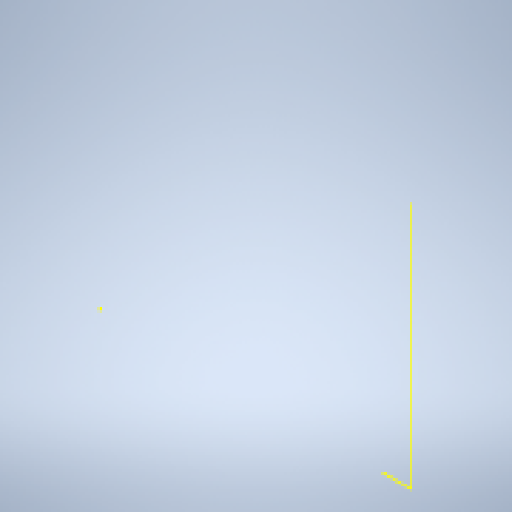
# Autodesk Inventor part: Soporte Motor
Saved by Autodesk Inventor 2024 (Build 280153000, 153)
## iProperties
Created: 2025-03-08
Part Number: Soporte Motor
Material: Genérico
Document SubType Name: Modeling
Designer: sergi
Density: 1 g/cm^3
Appearance: Valor por defecto
Author: sergi
Autodesk Inventor part; units mm, degrees
ref_plane "YZ Plane" through (0, 0, 0) normal (1, 0, 0) x (0, 1, 0)
ref_plane "XZ Plane" through (0, 0, 0) normal (0, 1, 0) x (-1, 0, 0)
ref_plane "XY Plane" through (0, 0, 0) normal (0, 0, 1) x (1, 0, 0)
sketch "Boceto1" plane through (0, 0, 0) normal (0, 0, 1) x (1, 0, 0)
  line L0 (42.301, 0) -> (42.301, 9.6) projected
  line L1 (42.302, 9.6) -> (42.302, 26.1) projected
  line L2 (42.301, 26.1) -> (42.301, 33.75) projected
  line L3 (38.301, 0) -> (42.301, 0) projected
  line L4 (4.001, 33.75) -> (38.301, 33.75) projected
  line L5 (38.301, 33.75) -> (42.301, 33.75) projected
  line L6 (0.001, 33.75) -> (4.001, 33.75) projected
  line L7 (0.001, 26.1) -> (0.001, 33.75) projected
  line L8 (0.001, 9.6) -> (0.001, 26.1) projected
  line L9 (0.001, 0) -> (0.001, 9.6) projected
  line L10 (42.301, 33.75) -> (0.001, 33.75)
  line L11 (0.001, 33.75) -> (0.001, 0)
  line L12 (0.001, 0) -> (42.301, 0)
  line L13 (42.301, 0) -> (42.301, 33.75)
  line L14 (42.501, 33.95) -> (-0.199, 33.95)
  line L15 (-0.199, 33.95) -> (-0.199, -0.2)
  line L16 (-0.199, -0.2) -> (42.501, -0.2)
  line L17 (42.501, -0.2) -> (42.501, 33.95)
  line L18 (42.501, 36.95) -> (-3.199, 36.95)
  line L19 (-3.199, 36.95) -> (-3.199, 0)
  line L20 (-3.199, -3.2) -> (45.501, -3.2)
  line L21 (45.501, 0) -> (45.501, 36.95)
  line L22 (42.301, 0) -> (45.501, 0)
  line L23 (0.001, 0) -> (-3.199, 0)
  line L24 (42.501, 33.95) -> (42.501, 36.95)
  point P0 (0, 0)
  point P1 (-0.199, 0)
  dimension "d0" = 0.2
  dimension "d1" = 3
  constraints: 30 end point, 6 parallel, 4 perpendicular, 2 point on line, 1 horizontal, 3 other
  measures "d0" distance between parallel lines of L13 L17
  measures "d1" distance between parallel lines of L17 L21
extrude "Extrusión1" add sketch "Boceto1" along normal blind 45.502 contours L14 L15 L23 L19 L18 L24
sketch "Boceto2" plane through (-0.199, 33.95, 0) normal (0, -1, 0) x (1, 0, 0)
  line L0 (0, 0) -> (42.7, 0) projected
  line L1 (42.7, 0) -> (42.7, 45.502) projected
  line L2 (0, 45.502) -> (42.7, 45.502) projected
  line L3 (0, 0) -> (0, 45.502) projected
  line L4 (42.7, 45.502) -> (0, 45.502)
  line L5 (0, 45.502) -> (0, 42.502)
  line L6 (0, 42.502) -> (42.7, 42.502)
  line L7 (42.7, 42.502) -> (42.7, 45.502)
  point P0 (0.199, 0)
  dimension "d4" = 3
  constraints: 8 end point, 2 parallel, 1 horizontal, 1 perpendicular, 1 point on line
  measures "d4" distance of L5.end L4.end
extrude "Extrusión2" add sketch "Boceto2" along normal up to surface (33.95 mm away) contours L3 L2 L1 L6
sketch "Boceto3" plane through (0, 0, 45.502) normal (0, 0, 1) x (1, 0, 0)
  line L0 (-3.199, 0) -> (42.501, 0) projected
  line L1 (42.501, 36.95) -> (42.501, 0) projected
  line L2 (42.501, 36.95) -> (-3.199, 36.95) projected
  line L3 (-3.199, 36.95) -> (-3.199, 0) projected
  line L4 (-6.5037, 43.25) -> (-6.5037, 58.25) projected
  line L5 (-6.5037, 43.25) -> (-6.5037, 58.25) projected
  line L6 (29.151, 9.6) -> (29.151, 3.2) projected
  line L7 (29.151, 0) -> (29.151, 3.2) projected
  line L8 (13.651, 3.6) -> (13.651, 9.1) projected
  line L9 (13.151, 3.2) -> (13.151, 0) projected
  line L10 (13.151, 9.6) -> (13.151, 3.2) projected
  line L11 (29.151, 9.6) -> (13.151, 9.6) projected
  line L12 (11.151, 0) -> (11.151, 3.2)
  line L13 (11.151, 3.2) -> (11.151, 11.6)
  line L14 (11.151, 11.6) -> (31.151, 11.6)
  line L15 (31.151, 11.6) -> (31.151, 3.2)
  line L16 (31.151, 3.2) -> (31.151, 0)
  point P0 (0, 0)
  point P1 (-15.9908, 43.25)
  dimension "d7" = 2
  constraints: 10 end point, 5 other
  measures "d7" distance between parallel lines of L11 L14
extrude "Extrusión3" cut sketch "Boceto3" against normal blind 10 contours L12 L13 L14 L15 L16 L0 L7 L6 L11 L10 L9 | L9 L10 L11 L6 L7 L0
sketch "Boceto4" plane through (-3.199, 36.95, 0) normal (0, 1, 0) x (1, 0, 0)
  circle A0 centre (24.35, -21.151) radius 2.5 projected
  circle A1 centre (24.35, -21.151) radius 15
  point P0 (3.199, 0)
  dimension "d10" = 30
  constraints: 1 centre point, 1 coincident
  measures "d10" diameter of A1
extrude "Extrusión4" cut sketch "Boceto4" against normal blind 10 contours A0 | A1
sketch "Boceto5" plane through (-3.199, 36.95, 0) normal (0, 1, 0) x (1, 0, 0)
  circle A0 centre (24.35, -21.151) radius 15 projected
  line L0 (45.7, 0) -> (0, 0) projected
  line L1 (0, 0) -> (0, -45.502) projected
  line L2 (45.7, -45.502) -> (0, -45.502) projected
  line L3 (45.7, 0) -> (45.7, -45.502) projected
  circle A1 centre (24.35, -21.151) radius 15 projected
  line L4 (45.7, -42.502) -> (3, -42.502) projected
  line L5 (3, 0) -> (3, -42.502) projected
  line L6 (3, 0) -> (45.7, 0) projected
  line L7 (45.7, 0) -> (45.7, -42.502) projected
  circle A2 centre (8.85, -36.651) radius 1.5 projected
  circle A3 centre (8.85, -5.651) radius 1.5 projected
  circle A4 centre (39.85, -5.6509) radius 1.5001 projected
  circle A5 centre (39.8499, -36.6509) radius 1.4998 projected
  circle A6 centre (39.8499, -36.6509) radius 2
  circle A7 centre (39.85, -5.6509) radius 2
  circle A8 centre (8.85, -5.651) radius 2
  circle A9 centre (8.85, -36.651) radius 2
  point P0 (3.199, 0)
  dimension "d13" = 4
  dimension "d14" = 4
  dimension "d15" = 4
  dimension "d16" = 4
  constraints: 4 centre point, 4 coincident
  measures "d13" diameter of A6
  measures "d14" diameter of A7
  measures "d15" diameter of A8
  measures "d16" diameter of A9
hole "Agujero1" at (5.651, 36.95, 36.651) at (5.651, 36.95, 5.651) at (36.651, 36.95, 5.6509) at (36.6509, 36.95, 36.6509) direction (0, -1, 0) diameter 3.5 end through all
sketch "Boceto6" plane through (0, 0, 45.502) normal (0, 0, 1) x (1, 0, 0)
  line L0 (31.151, 11.6) -> (31.151, 0) projected
  line L1 (31.151, 0) -> (42.501, 0) projected
  line L2 (42.501, 36.95) -> (42.501, 0) projected
  line L3 (42.501, 36.95) -> (-3.199, 36.95) projected
  line L4 (-3.199, 36.95) -> (-3.199, 0) projected
  line L5 (-3.199, 0) -> (11.151, 0) projected
  line L6 (11.151, 0) -> (11.151, 11.6) projected
  line L7 (11.151, 11.6) -> (31.151, 11.6) projected
  line L8 (42.501, 36.95) -> (39.501, 36.95)
  line L9 (39.501, 36.95) -> (39.501, 0)
  line L10 (39.501, 0) -> (42.501, 0)
  line L11 (42.501, 0) -> (42.501, 36.95)
  point P0 (0, 0)
  dimension "d24" = 3
  constraints: 8 end point, 2 parallel, 1 horizontal, 1 perpendicular, 1 point on line
  measures "d24" distance of L10.end L9.end
extrude "Extrusión5" add sketch "Boceto6" along normal blind 10 contours L9 L3 L2 L1
fillet "Empalme1" radius 3 1 edges at (39.501, 18.475, 45.502)
sketch "Boceto7" plane through (39.501, 0, 55.502) normal (-1, 0, 0) x (0, 0, 1)
  line L0 (-7, 0) -> (-7, 36.95) projected
  line L1 (-7, 0) -> (0, 0) projected
  line L2 (0, 36.95) -> (0, 0) projected
  line L3 (-7, 36.95) -> (0, 36.95) projected
  line L4 (-7, 36.95) -> (0, 36.95)
  line L5 (0, 36.95) -> (0, 29.95)
  line L6 (0, 29.95) -> (-7, 29.95)
  line L7 (-7, 29.95) -> (-7, 36.95)
  line L8 (-55.502, 36.95) -> (0, 36.95) projected
  line L9 (-7, 29.95) -> (0, 36.95)
  circle A0 centre (-3.5, 33.45) radius 2
  line L10 (-7, 0) -> (0, 0)
  line L11 (0, 0) -> (0, 7)
  line L12 (0, 7) -> (-7, 7)
  line L13 (-7, 7) -> (-7, 0)
  line L14 (-7, 0) -> (0, 7)
  circle A1 centre (-3.5, 3.5) radius 2
  point P0 (-55.502, 0)
  dimension "d28" = 7
  dimension "d29" = 4
  dimension "d30" = 7
  dimension "d31" = 7
  dimension "d32" = 4
  constraints: 20 end point, 4 parallel, 2 centre point, 2 horizontal, 2 midpoint, 2 perpendicular, 1 point on line
  measures "d28" distance of L4.end L5.end
  measures "d29" diameter of A0
  measures "d30" distance of L12.end L11.end
  measures "d31" distance of L11.end L10.end
  measures "d32" diameter of A1
hole "Agujero2" at (39.501, 33.45, 52.002) at (39.501, 3.5, 52.002) direction (1, 0, 0) diameter 3.5 end through all
sketch "Boceto8" plane through (-3.199, 0, 0) normal (-1, 0, 0) x (0, 0, 1)
  line L0 (0, 36.95) -> (0, 0) projected
  line L1 (0, 0) -> (45.502, 0) projected
  line L2 (45.502, 36.95) -> (45.502, 0) projected
  line L3 (0, 36.95) -> (45.502, 36.95) projected
  line L4 (0, 0) -> (3, 0)
  line L5 (3, 0) -> (3, 36.95)
  line L6 (3, 36.95) -> (0, 36.95)
  line L7 (0, 36.95) -> (0, 0)
  point P0 (0, 0)
  dimension "d40" = 3
  constraints: 8 end point, 2 parallel, 1 horizontal, 1 perpendicular, 1 point on line
  measures "d40" distance of L6.end L5.end
extrude "Extrusión6" add sketch "Boceto8" along normal blind 10 contours L3 L5 L1 L0
fillet "Empalme2" radius 3 1 edges at (-3.199, 18.475, 3)
sketch "Boceto9" plane through (-13.199, 0, 3) normal (0, 0, 1) x (1, 0, 0)
  line L0 (7, 36.95) -> (7, 0) projected
  line L1 (7, 36.95) -> (0, 36.95) projected
  line L2 (0, 0) -> (0, 36.95) projected
  line L3 (7, 0) -> (0, 0) projected
  line L4 (0, 36.95) -> (7, 36.95)
  line L5 (7, 36.95) -> (7, 29.95)
  line L6 (7, 29.95) -> (0, 29.95)
  line L7 (0, 29.95) -> (0, 36.95)
  line L8 (0, 0) -> (7, 0)
  line L9 (7, 0) -> (7, 7)
  line L10 (7, 7) -> (0, 7)
  line L11 (0, 7) -> (0, 0)
  line L12 (0, 29.95) -> (7, 36.95)
  line L13 (0, 7) -> (7, 0)
  circle A0 centre (3.5, 33.45) radius 1.75
  circle A1 centre (3.5, 3.5) radius 1.75
  point P0 (13.199, 0)
  dimension "d44" = 7
  dimension "d45" = 7
  dimension "d46" = 7
  dimension "d47" = 3.5
  dimension "d48" = 3.5
  constraints: 20 end point, 4 parallel, 2 centre point, 2 horizontal, 2 midpoint, 2 perpendicular, 1 point on line
  measures "d44" distance of L4.end L5.end
  measures "d45" distance of L10.end L9.end
  measures "d46" distance of L9.end L8.end
  measures "d47" diameter of A0
  measures "d48" diameter of A1
hole "Agujero3" at (-9.699, 33.45, 3) at (-9.699, 3.5, 3) direction (0, 0, -1) diameter 3.5 end through all
fillet "Empalme3" radius 3 1 edges at (-3.199, 18.475, 45.502)
